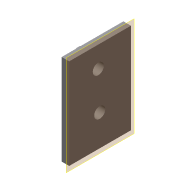
# Autodesk Inventor part: GearBoxLid2
Saved by Autodesk Inventor 2018 (Build 220112000, 112)
## iProperties
Created: 2018-10-26
Part Number: GearBoxLid2
Material: Generic
Document SubType Name: Modeling
Designer: Vulnic
Density: 1 g/cm^3
Appearance: Default
Author: Vulnic
Autodesk Inventor part; units mm, degrees
ref_plane "YZ Plane" through (0, 0, 0) normal (1, 0, 0) x (0, 1, 0)
ref_plane "XZ Plane" through (0, 0, 0) normal (0, 1, 0) x (-1, 0, 0)
ref_plane "Work Plane1" through (25.2802, 41.8518, -22.309) normal (1, 0, 0) x (0, 1, 0)
sketch "Sketch1" plane through (25.2802, 41.8518, -22.309) normal (1, 0, 0) x (0, 1, 0)
  line L0 (12.4048, 23.6333) -> (-12.1268, 23.6333) projected
  line L1 (-12.1268, 23.6333) -> (-12.1268, -12.3269) projected
  line L2 (12.4048, -12.3269) -> (12.4048, 23.6333) projected
  line L3 (-12.1268, -12.3269) -> (12.4048, -12.3269) projected
  circle A0 centre (0, 0) radius 2.2
  circle A1 centre (-0.5578, 15.2966) radius 2.2
  line L4 (12.4048, 23.6333) -> (-12.1268, 23.6333)
  line L5 (-12.1268, 23.6333) -> (-12.1268, -12.3269)
  line L6 (-12.1268, -12.3269) -> (12.4048, -12.3269)
  line L7 (12.4048, -12.3269) -> (12.4048, 23.6333)
  circle A2 centre (-0.569, 15.3293) radius 3.5 projected
  circle A3 centre (0, 0) radius 3.2587 projected
  point P0 (-41.8518, 22.309)
  constraints: 8 end point, 2 centre point, 2 parallel, 1 horizontal, 1 perpendicular
extrude "Extrusion1" add sketch "Sketch1" against normal blind 3 contours L2 L3 L1 L0 | A1
sketch "Sketch2" plane through (25.2802, 41.8518, -22.309) normal (1, 0, 0) x (0, 0, -1)
  circle A0 centre (-15.2966, -0.5578) radius 2.2
  circle A1 centre (0, 0) radius 2.2
  circle A2 centre (-15.3293, -0.569) radius 3.5 projected
  circle A3 centre (-15.3293, -0.569) radius 3.5
  circle A4 centre (0, 0) radius 3.2587
  point P0 (-22.309, -41.8518)
  constraints: 4 centre point, 2 coincident, 1 concentric
extrude "Extrusion2" add sketch "Sketch2" against normal blind 6
body "Solid1"
